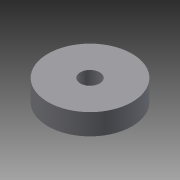
# Autodesk Inventor part: body-back
Saved by Autodesk Inventor 2013 (Build 170138000, 138)
## iProperties
Created: 2012-09-08
Part Number: body-back
Material: Generic
Document SubType Name: Modeling
Designer: frankenteddy
Density: 1 g/cm^3
Author: frankenteddy
Autodesk Inventor part; units mm, degrees
ref_plane "YZ Plane" through (0, 0, 0) normal (1, 0, 0) x (0, 1, 0)
ref_plane "XZ Plane" through (0, 0, 0) normal (0, 1, 0) x (-1, 0, 0)
ref_plane "XY Plane" through (0, 0, 0) normal (0, 0, 1) x (1, 0, 0)
sketch "Sketch1" plane through (0, 0, 0) normal (0, 0, 1) x (1, 0, 0)
  line L0 (-92.7646, -8.503) -> (-89.7646, -8.503)
  line L1 (-89.7646, -8.503) -> (-89.7646, -11.753)
  line L2 (-89.7646, -11.753) -> (-92.7646, -11.753)
  line L3 (-92.7646, -11.753) -> (-92.7646, -8.503)
  line L4 (-92.7646, -21.6527) -> (-89.7646, -21.6527)
  line L5 (-89.7646, -21.6527) -> (-89.7646, -21.7527)
  line L6 (-89.7646, -21.7527) -> (-92.7646, -21.7527)
  line L7 (-92.7646, -21.7527) -> (-92.7646, -21.6527)
  circle A0 centre (-35.0617, 15.7002) radius 6.5
  circle A1 centre (-35.0617, 15.7002) radius 1.5
  point P0 (0, 0)
  dimension "d3" = 3
  dimension "mat" = 3.25
  dimension "d5" = 3
  dimension "kerf" = 0.1
  dimension "d35" = 13
  dimension "d36" = 3
  constraints: 16 end point, 4 parallel, 2 centre point, 2 horizontal, 2 perpendicular, 1 coincident
  measures "d3" distance of L1.end L2.end
  measures "mat" distance of L0.end L1.end
  measures "d5" distance of L5.end L6.end
  measures "kerf" distance of L4.end L5.end
  measures "d35" diameter of A0
  measures "d36" diameter of A1
extrude "Extrusion5" add sketch "Sketch1" along normal blind 3.25 contours A0
equation "\"d37\" = mat"
body "Solid3"
